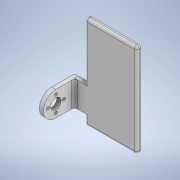
# Autodesk Inventor part: GripperConstant
Saved by Autodesk Inventor 2020 (Build 240168000, 168)
## iProperties
Created: 2019-12-26
Part Number: GripperConstant
Material: Generic
Document SubType Name: Modeling
Designer: tdmp4
Density: 1 g/cm^3
Appearance: Default
Author: tdmp4
Autodesk Inventor part; units mm, degrees
ref_plane "YZ Plane" through (0, 0, 0) normal (1, 0, 0) x (0, 1, 0)
ref_plane "XZ Plane" through (0, 0, 0) normal (0, 1, 0) x (-1, 0, 0)
ref_plane "XY Plane" through (0, 0, 0) normal (0, 0, 1) x (1, 0, 0)
sketch "Sketch1" plane through (0, 0, 0) normal (1, 0, 0) x (0, 1, 0)
  circle A0 centre (0, 0) radius 15.24
  circle A1 centre (9.779, 0) radius 1.7859
  circle A2 centre (0, -9.779) radius 1.7859
  circle A3 centre (-9.779, 0) radius 1.7859
  circle A4 centre (0, 9.779) radius 1.7859
  circle A5 centre (0, 0) radius 6.35
  arc A6 (-1.7785, -9.6159) -> (1.7785, -9.6159) centre (0, 0) ccw
  dimension "d0" = 30.48
  dimension "d2" = 3.5719
  dimension "d3" = 3.5719
  dimension "d4" = 3.5719
  dimension "d5" = 3.5719
  dimension "d6" = 12.7
  constraints: 7 centre point, 5 point on circle, 3 coincident
  measures "d0" diameter of A0
  measures "d2" diameter of A1
  measures "d3" diameter of A2
  measures "d4" diameter of A3
  measures "d5" diameter of A4
  measures "d6" diameter of A5
extrude "Extrusion1" add sketch "Sketch1" along normal blind 5.08
sketch "Sketch5" plane through (5.08, 0, 0) normal (1, 0, 0) x (0, 0, -1)
  circle A0 centre (0, 0) radius 15.24 projected
  arc A1 (0, -15.24) -> (0, 15.24) centre (0, 0) ccw
  line L0 (0, 15.24) -> (27.94, 15.24)
  line L1 (27.94, 15.24) -> (27.94, -15.24)
  line L2 (27.94, -15.24) -> (0, -15.24)
  dimension "d17" = 27.94
  dimension "d18" = 30.48
  constraints: 6 end point, 4 point on circle, 2 tangent, 1 centre point, 1 horizontal, 1 perpendicular, 1 vertical
  measures "d17" distance of L0.start L0.end
  measures "d18" distance of L0.end L1.end
extrude "Extrusion3" add sketch "Sketch5" against normal blind 5.08 contours A0 L0 L1 L2
sketch "Sketch6" plane through (5.08, 0, 0) normal (1, 0, 0) x (0, 0, -1)
  line L0 (27.94, -15.24) -> (27.94, 15.24) projected
  line L1 (27.94, -15.24) -> (22.86, -15.24)
  line L2 (22.86, -15.24) -> (22.86, 15.6141)
  line L3 (22.86, 15.6141) -> (27.94, 15.6141)
  line L4 (27.94, 15.6141) -> (27.94, -15.24)
  point P0 (0, 0)
  dimension "d21" = 5.08
  constraints: 8 end point, 2 parallel, 1 horizontal, 1 perpendicular
  measures "d21" distance of L2.end L3.end
extrude "Extrusion4" add sketch "Sketch6" along normal blind 12.7
sketch "Sketch7" plane through (0, -15.24, -27.94) normal (0, 0, -1) x (-1, 0, 0)
  line L0 (-17.78, 30.8541) -> (-17.78, 0) projected
  line L1 (-17.78, 0) -> (-81.28, 0)
  line L2 (-81.28, 0) -> (-81.28, 101.6)
  line L3 (-81.28, 101.6) -> (-17.78, 101.6)
  line L4 (-17.78, 101.6) -> (-17.78, 0)
  line L5 (-5.08, 0) -> (-17.78, 0) projected
  line L6 (-17.78, 0) -> (-81.28, 0)
  line L7 (-81.28, 0) -> (-81.28, -12.7)
  line L8 (-81.28, -12.7) -> (-17.78, -12.7)
  line L9 (-17.78, -12.7) -> (-17.78, 0)
  point P0 (0, 15.24)
  dimension "d24" = 63.5
  dimension "d25" = 101.6
  dimension "d26" = 12.7
  constraints: 16 end point, 4 parallel, 2 horizontal, 2 perpendicular
  measures "d24" distance of L2.end L3.end
  measures "d25" distance of L1.end L2.end
  measures "d26" distance of L6.end L7.end
extrude "Extrusion5" add sketch "Sketch7" against normal blind 5.08
fillet "Fillet1" radius 3.175 11 edges at (5.08, 0, -22.86) (17.78, 86.36, -25.4) (81.28, 86.36, -25.4) (81.28, -27.94, -25.4) (0, 0, -27.94) (17.78, -27.94, -25.4) (49.53, -27.94, -22.86) (17.78, -21.59, -22.86) (17.78, 50.987, -22.86) (49.53, 86.36, -22.86) (81.28, 29.21, -22.86)
body "Solid1"
